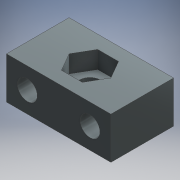
# Autodesk Inventor part: back_sprocket_holder
Saved by Autodesk Inventor 2016 (Build 200138000, 138)
## iProperties
Created: 2017-01-06
Part Number: back_sprocket_holder
Material: Generic
Document SubType Name: Modeling
Designer: hesaon
Density: 1 g/cm^3
Appearance: Default
Author: hesaon
Autodesk Inventor part; units mm, degrees
ref_plane "YZ Plane" through (0, 0, 0) normal (1, 0, 0) x (0, 1, 0)
ref_plane "XZ Plane" through (0, 0, 0) normal (0, 1, 0) x (-1, 0, 0)
ref_plane "XY Plane" through (0, 0, 0) normal (0, 0, 1) x (1, 0, 0)
sketch "Sketch1" plane through (0, 0, 0) normal (0, 1, 0) x (-1, 0, 0)
  line L0 (0, 0) -> (30, 0)
  line L1 (30, 0) -> (30, -12)
  line L2 (30, -12) -> (0, -12)
  line L3 (0, -12) -> (0, 0)
  circle A0 centre (24, -6) radius 2.85
  circle A1 centre (6, -6) radius 2.85
  dimension "d0" = 30
  dimension "d1" = 12
  dimension "d2" = 5.7
  dimension "d3" = 5.7
  dimension "d4" = 6
  dimension "d5" = 18
  dimension "d6" = 6
  constraints: 8 end point, 2 centre point, 2 parallel, 1 horizontal, 1 horizontal alignment, 1 perpendicular
  measures "d0" distance of L1.end L2.end
  measures "d1" distance of L0.end L1.end
  measures "d2" diameter of A0
  measures "d3" diameter of A1
  measures "d4" distance from line of L1 A0.centre
  measures "d5" distance of A1.centre A0.centre
  measures "d6" distance from line of L2 A0.centre
extrude "Extrusion1" add sketch "Sketch1" along normal blind 18
sketch "Sketch2" plane through (-30, 0, 0) normal (0, 0, 1) x (1, 0, 0)
  line L0 (21.0044, 9) -> (18.0022, 3.8)
  line L1 (18.0022, 3.8) -> (11.9978, 3.8)
  line L2 (11.9978, 3.8) -> (8.9956, 9)
  line L3 (8.9956, 9) -> (11.9978, 14.2)
  line L4 (11.9978, 14.2) -> (18.0022, 14.2)
  line L5 (18.0022, 14.2) -> (21.0044, 9)
  line L6 (0, 18) -> (30, 18) projected
  line L7 (30, 0) -> (30, 18) projected
  point P0 (15, 9)
  dimension "d9" = 10.4
  dimension "d10" = 9
  dimension "d11" = 15
  constraints: 12 end point, 1 parallel, 13 other
  measures "d9" distance between parallel lines of L1 L4
  measures "d10" distance from line of L6 point (15, 9)
  measures "d11" distance from line of L7 point (15, 9)
extrude "Extrusion2" cut sketch "Sketch2" against normal blind 5
sketch "Sketch4" plane through (0, 0, -12) normal (0, 0, -1) x (-1, 0, 0)
  circle A0 centre (15, 9) radius 3
  line L0 (30, 0) -> (0, 0) projected
  line L1 (0, 0) -> (0, 18) projected
  dimension "d14" = 6
  dimension "d15" = 9
  dimension "d16" = 15
  constraints: 1 centre point
  measures "d14" diameter of A0
  measures "d15" distance from line of L0 A0.centre
  measures "d16" distance from line of L1 A0.centre
extrude "Extrusion3" cut sketch "Sketch4" against normal through all
body "Solid1"
